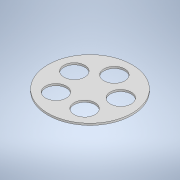
# Autodesk Inventor part: filterHolder
Saved by Autodesk Inventor 2021 (Build 250183000, 183)
## iProperties
Created: 2020-04-12
Part Number: filterHolder
Material: Generic
Document SubType Name: Modeling
Designer: robst
Density: 1 g/cm^3
Appearance: Default
Author: robst
Autodesk Inventor part; units mm, degrees
ref_plane "YZ Plane" through (0, 0, 0) normal (1, 0, 0) x (0, 1, 0)
ref_plane "XZ Plane" through (0, 0, 0) normal (0, 1, 0) x (-1, 0, 0)
ref_plane "XY Plane" through (0, 0, 0) normal (0, 0, 1) x (1, 0, 0)
sketch "Sketch1" plane through (0, 0, 0) normal (0, 1, 0) x (-1, 0, 0)
  circle A0 centre (0, 0) radius 57.4978
  circle A1 centre (0, 0) radius 33.3678 construction
  circle A2 centre (0, -33.3678) radius 14.2875
  circle A3 centre (31.7347, -10.3112) radius 14.2875
  circle A4 centre (19.6131, 26.9951) radius 14.2875
  circle A5 centre (-19.6131, 26.9951) radius 14.2875
  circle A6 centre (-31.7347, -10.3112) radius 14.2875
  dimension "wheelFilterDiameter" = 66.7357
  dimension "wheelOuterDiameter" = 114.9957
  dimension "filterThreadDiameter" = 28.575
  dimension "d5" = 360
  constraints: 6 centre point, 2 coincident, 1 vertical alignment, 13 other
  measures "wheelOuterDiameter" diameter of A0
  measures "filterThreadDiameter" diameter of A2
extrude "Extrusion1" add sketch "Sketch1" against normal blind 2.54
equation "\"wheelFilterDiameter\" = 0.318471 * wheelFilterCircumference"
equation "\"wheelOuterDiameter\" = filterDiameter + wheelFilterDiameter + 2 * distanceFromFilterToEdge"
equation "\"distanceBetweenFilters\" = 12.7"
equation "\"distanceFromFilterToEdge\" = 9.525"
equation "\"filterDiameter\" = 29.21"
equation "\"wheelFilterCircumference\" = 209.55"
body "Solid1"
